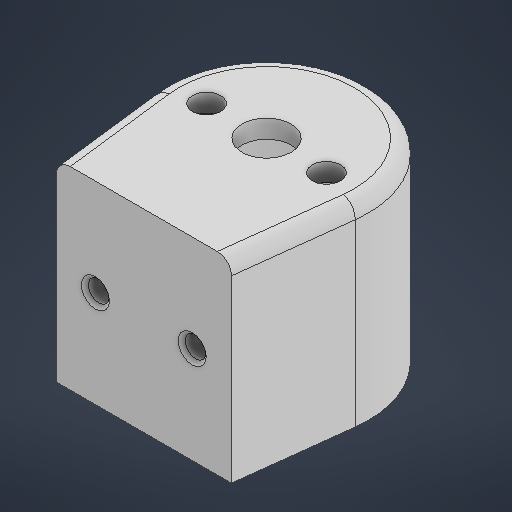
# Autodesk Inventor part: motor_holder
Saved by Autodesk Inventor 2027 (Build 310192000, 192)
## iProperties
Created: 2026-05-11
Part Number: motor_holder
Material: Generic
Document SubType Name: Modeling
Designer: maksi
Density: 1 g/cm^3
Appearance: Default
Author: maksi
Autodesk Inventor part; units mm, degrees
ref_plane "YZ Plane" through (0, 0, 0) normal (1, 0, 0) x (0, 1, 0)
ref_plane "XZ Plane" through (0, 0, 0) normal (0, 1, 0) x (-1, 0, 0)
ref_plane "XY Plane" through (0, 0, 0) normal (0, 0, 1) x (1, 0, 0)
sketch "Sketch1" plane through (0, 0, 0) normal (0, 1, 0) x (-1, 0, 0)
  circle A0 centre (-8.5046, 0.0113) radius 2
  circle A1 centre (0.0454, 0.0113) radius 12.5
  circle A2 centre (-8.5046, 0.0113) radius 1.5
  circle A3 centre (8.5954, 0.0113) radius 2
  circle A4 centre (8.5954, 0.0113) radius 1.5
  circle A5 centre (0.0454, 0.0113) radius 3.5
  line L0 (-12.4546, 0.0113) -> (12.5454, 0.0113)
  line L1 (12.5454, 17.5113) -> (-12.4546, 17.5113)
  circle A6 centre (0.0454, 0.0113) radius 14.5
  line L2 (-12.4546, 17.5113) -> (-14.3509, 1.7426)
  line L3 (12.5454, 17.5113) -> (14.4417, 1.7426)
  circle A7 centre (0.0454, 0.0113) radius 12.8
  point P0 (0, 0)
  dimension "d0" = 17.5
  dimension "d2" = 2
  dimension "d5" = 0.3
  constraints: 8 centre point, 8 end point, 4 point on circle, 2 tangent, 1 horizontal, 1 parallel
  measures "d0" distance of L1.start L0.end
  measures "d2" radial gap between concentric circles of A1 A6
  measures "d5" radial gap between concentric circles of A1 A7
extrude "Extrusion1" add sketch "Sketch1" along normal blind 2.6 contours L0 A5 A3 A1 A0 | A0 L0 A1 A3 A5 | L3 A6 L2 L1 | A6 | A7
extrude "Extrusion2" add sketch "Sketch1" against normal blind 25 contours L3 A6 L2 L1 | A6
sketch "Sketch2" plane through (-12.5454, 2.6, 17.5113) normal (0, 0, 1) x (1, 0, 0)
  line L0 (25, -27.6) -> (0, -27.6) construction
  line L1 (25, -27.6) -> (0, 0) construction
  line L2 (0, -27.6) -> (25, 0) construction
  line L3 (27, 0) -> (-2, 0) construction
  line L4 (19.4, -13.8) -> (5.6, -13.8) construction
  point P0 (12.5454, -2.6)
  point P1 (26.8963, 0)
  point P2 (-1.8963, 0)
  point P3 (12.5, -13.8)
  dimension "d8" = 13.8
  constraints: 6 end point, 2 midpoint, 1 horizontal, 1 point on line
  measures "d8" distance of L4.start L4.end
hole "Hole1" at (6.8546, -11.2, 17.5113) at (-6.9454, -11.2, 17.5113) direction (0, 0, -1) diameter 3 depth 12 tip angle 118 countersink diameter 4 countersink angle 90
fillet "Fillet1" radius 2 3 edges at (-0.0454, 2.6, -14.4887) (-13.4935, 2.6, 9.627) (13.4027, 2.6, 9.627)
body "Solid1"
